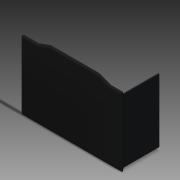
# Autodesk Inventor part: Simple3DPrintBackplate01
Saved by Autodesk Inventor 2015 (Build 190159000, 159)
## iProperties
Created: 2015-09-24
Part Number: Simple3DPrintBackplate01
Material: Aluminum 6061 Black Anodized
Document SubType Name: Modeling
Designer: -
Density: 2.71 g/cm^3
Appearance: Aluminum - Flat - Version 1.1
Author: -
Autodesk Inventor part; units mm, degrees
ref_plane "YZ Plane" through (0, 0, 0) normal (1, 0, 0) x (0, 1, 0)
ref_plane "XZ Plane" through (0, 0, 0) normal (0, 1, 0) x (-1, 0, 0)
ref_plane "XY Plane" through (0, 0, 0) normal (0, 0, 1) x (1, 0, 0)
sketch "Sketch1" plane through (0, 0, 0) normal (0, 0, 1) x (1, 0, 0)
  line L0 (25.1473, 47.4388) -> (-25.1473, 47.4388)
  line L1 (-25.8314, 47.3182) -> (-38.1686, 42.8278)
  line L2 (-38.8527, 42.7072) -> (-53.924, 42.7072)
  line L3 (-55.924, 40.7072) -> (-55.924, -28.8108)
  line L4 (-53.924, -30.8108) -> (62.994, -30.8108)
  line L5 (64.994, -28.8108) -> (64.994, 40.7072)
  line L6 (62.994, 42.7072) -> (38.8527, 42.7072)
  line L7 (38.1686, 42.8278) -> (25.8314, 47.3182)
  line L8 (0, 0) -> (0, 61.2972) construction
  arc A0 (64.994, 40.7072) -> (62.994, 42.7072) centre (62.994, 40.7072) ccw
  arc A1 (62.994, -30.8108) -> (64.994, -28.8108) centre (62.994, -28.8108) ccw
  arc A2 (-55.924, -28.8108) -> (-53.924, -30.8108) centre (-53.924, -28.8108) ccw
  arc A3 (-53.924, 42.7072) -> (-55.924, 40.7072) centre (-53.924, 40.7072) ccw
  arc A4 (-38.8527, 42.7072) -> (-38.1686, 42.8278) centre (-38.8527, 44.7072) ccw
  arc A5 (-25.1473, 47.4388) -> (-25.8314, 47.3182) centre (-25.1473, 45.4388) ccw
  arc A6 (25.8314, 47.3182) -> (25.1473, 47.4388) centre (25.1473, 45.4388) ccw
  arc A7 (38.1686, 42.8278) -> (38.8527, 42.7072) centre (38.8527, 44.7072) ccw
  point P0 (25.5, 47.4388)
  point P1 (-25.5, 47.4388)
  point P2 (-38.5, 42.7072)
  point P3 (-55.924, 42.7072)
  point P4 (-55.924, -30.8108)
  point P5 (64.994, 42.7072)
  point P6 (38.5, 42.7072)
  point P7 (0, 47.4388)
  dimension "d48" = 51
  dimension "d50" = 160
  dimension "d51" = 160
  dimension "d52" = 13
  dimension "d53" = 17.424
  dimension "d54" = 26.494
  dimension "d55" = 73.518
  dimension "d56" = 13
  dimension "d57" = 2
  constraints: 18 end point, 16 point on circle, 16 point on line, 16 tangent, 8 centre point, 7 equal radius, 4 perpendicular, 2 horizontal, 1 midpoint, 1 parallel, 1 vertical, 1 other
  measures "d48" distance of point (25.5, 47.439) point (-25.5, 47.439)
  measures "d50" angle of L0 L7
  measures "d51" angle of L0 L1
  measures "d52" horizontal distance of point (-38.5, 42.707) point (-25.5, 47.439)
  measures "d53" distance of point (-38.5, 42.707) point (-55.924, 42.707)
  measures "d54" distance of point (64.994, 42.707) point (38.5, 42.707)
  measures "d55" distance of point (-55.924, 42.707) point (-55.924, -30.811)
  measures "d56" horizontal distance of point (25.5, 47.439) point (38.5, 42.707)
  measures "d57" radius of A0
extrude "Extrusion1" add sketch "Sketch1" along normal blind 2
chamfer "Chamfer1" distance 1.5 distance2 1 16 edges at (50.9233, 42.7072, 2) (38.5054, 42.7376, 2) (32, 45.073, 2) (25.4946, 47.4084, 2) (0, 47.4388, 2) (-25.4946, 47.4084, 2) (-32, 45.073, 2) (-38.5054, 42.7376, 2) (-46.3883, 42.7072, 2) (-55.3382, 42.1214, 2) (-55.924, 5.9482, 2) (-55.3382, -30.225, 2) (4.535, -30.8108, 2) (64.4082, -30.225, 2) (64.994, 5.9482, 2) (64.4082, 42.1214, 2) measured on face at (64.0547, -29.8715, 2) measured on face at (64.0547, 41.7679, 2) measured on face at (-25.4078, 46.916, 2) measured on face at (31.829, 44.6032, 2) measured on face at (50.9233, 42.2072, 2) measured on face at (-38.4185, 42.2452, 2) measured on face at (-46.3883, 42.2072, 2) measured on face at (-55.424, 5.9482, 2) measured on face at (-31.829, 44.6032, 2) measured on face at (25.4078, 46.916, 2) measured on face at (4.535, -30.3108, 2) measured on face at (38.4185, 42.2452, 2) measured on face at (0, 46.9388, 2) measured on face at (64.494, 5.9482, 2) measured on face at (-54.9847, 41.7679, 2) measured on face at (-54.9847, -29.8715, 2)
fillet "Fillet1" radius 2 16 edges at (-54.2776, 41.0608, 2) (-46.3883, 41.2072, 2) (-38.2449, 41.2604, 2) (-31.487, 43.6635, 2) (-25.2342, 45.9312, 2) (0, 45.9388, 2) (25.2342, 45.9312, 2) (31.487, 43.6635, 2) (38.2449, 41.2604, 2) (50.9233, 41.2072, 2) (63.3476, 41.0608, 2) (63.494, 5.9482, 2) (63.3476, -29.1643, 2) (4.535, -29.3108, 2) (-54.2776, -29.1643, 2) (-54.424, 5.9482, 2)
fillet "Fillet2" radius 1 16 edges at (-55.3382, -30.225, 1) (4.535, -30.8108, 1) (64.4082, -30.225, 1) (64.994, 5.9482, 1) (64.4082, 42.1214, 1) (50.9233, 42.7072, 1) (38.5054, 42.7376, 1) (32, 45.073, 1) (25.4946, 47.4084, 1) (0, 47.4388, 1) (-25.4946, 47.4084, 1) (-32, 45.073, 1) (-38.5054, 42.7376, 1) (-46.3883, 42.7072, 1) (-55.3382, 42.1214, 1) (-55.924, 5.9482, 1)
feature "Lip1" [suppressed]
sketch "Sketch8" plane through (0, 0, 0) normal (0, 0, -1) x (-1, 0, 0)
  line L0 (-64.994, 40.7072) -> (-64.994, -28.8108) projected
  arc A0 (-64.994, -28.8108) -> (-62.994, -30.8108) centre (-62.994, -28.8108) ccw projected
  line L1 (-62.994, -30.8108) -> (53.924, -30.8108) projected
  arc A1 (53.924, -30.8108) -> (55.924, -28.8108) centre (53.924, -28.8108) ccw projected
  line L2 (55.924, -28.8108) -> (55.924, 40.7072) projected
  arc A2 (55.924, 40.7072) -> (53.924, 42.7072) centre (53.924, 40.7072) ccw projected
  line L3 (53.924, 42.7072) -> (38.8527, 42.7072) projected
  arc A3 (38.1686, 42.8278) -> (38.8527, 42.7072) centre (38.8527, 44.7072) ccw projected
  line L4 (38.1686, 42.8278) -> (25.8314, 47.3182) projected
  arc A4 (25.8314, 47.3182) -> (25.1473, 47.4388) centre (25.1473, 45.4388) ccw projected
  line L5 (25.1473, 47.4388) -> (-25.1473, 47.4388) projected
  arc A5 (-25.1473, 47.4388) -> (-25.8314, 47.3182) centre (-25.1473, 45.4388) ccw projected
  line L6 (-25.8314, 47.3182) -> (-38.1686, 42.8278) projected
  arc A6 (-38.8527, 42.7072) -> (-38.1686, 42.8278) centre (-38.8527, 44.7072) ccw projected
  line L7 (-38.8527, 42.7072) -> (-62.994, 42.7072) projected
  arc A7 (-62.994, 42.7072) -> (-64.994, 40.7072) centre (-62.994, 40.7072) ccw projected
  line L8 (-60.894, 40.6072) -> (-38.8527, 40.6072)
  arc A8 (-38.8527, 40.6072) -> (-37.4504, 40.8545) centre (-38.8527, 44.7072) ccw
  line L9 (-37.4504, 40.8545) -> (-25.7925, 45.0976)
  line L10 (-24.4244, 45.3388) -> (24.4244, 45.3388)
  line L11 (25.7925, 45.0976) -> (37.4504, 40.8545)
  arc A9 (37.4504, 40.8545) -> (38.8527, 40.6072) centre (38.8527, 44.7072) ccw
  line L12 (38.8527, 40.6072) -> (51.824, 40.6072)
  line L13 (53.824, 38.6072) -> (53.824, -26.7108)
  line L14 (51.824, -28.7108) -> (-60.894, -28.7108)
  line L15 (-62.894, -26.7108) -> (-62.894, 38.6072)
  arc A10 (-60.894, 40.6072) -> (-62.894, 38.6072) centre (-60.894, 38.6072) ccw
  arc A11 (-62.894, -26.7108) -> (-60.894, -28.7108) centre (-60.894, -26.7108) ccw
  arc A12 (51.824, -28.7108) -> (53.824, -26.7108) centre (51.824, -26.7108) ccw
  arc A13 (53.824, 38.6072) -> (51.824, 40.6072) centre (51.824, 38.6072) ccw
  arc A14 (-24.4244, 45.3388) -> (-25.7925, 45.0976) centre (-24.4244, 41.3388) ccw
  arc A15 (25.7925, 45.0976) -> (24.4244, 45.3388) centre (24.4244, 41.3388) ccw
  point P0 (0, 0)
  dimension "d62" = 2.1
  dimension "d63" = 2
  dimension "d64" = 4
  constraints: 16 end point, 16 point on circle, 12 tangent, 8 centre point, 4 equal radius, 9 other
  measures "d62" distance between parallel lines of L7 L8
  measures "d63" radius of A10
  measures "d64" radius of A14
extrude "Extrusion7" add sketch "Sketch8" along normal blind 1 contours L8 A8 L9 A14 L10 A15 L11 A9 L12 A13 L13 A12 L14 A11 L15 A10
sketch "Sketch4" plane through (0, 0, 2) normal (0, 0, 1) x (1, 0, 0)
  line L0 (92.6097, 61.0907) -> (51.0597, 61.0907)
  line L1 (51.0597, 61.0907) -> (51.0597, -62.6292)
  line L2 (51.0597, -62.6292) -> (92.6097, -62.6292)
  line L3 (92.6097, -62.6292) -> (92.6097, 61.0907)
  line L4 (64.5487, 40.7072) -> (64.5487, -28.8108) projected
  point P0 (0, 0)
  dimension "d21" = 123.7199
  dimension "d22" = 41.55
  dimension "d58" = 13.489
  constraints: 8 end point, 2 parallel, 1 horizontal, 1 perpendicular
  measures "d21" distance between parallel lines of L2 L0
  measures "d22" distance between parallel lines of L3 L1
  measures "d58" distance between parallel lines of L1 L4
extrude "Extrusion3" cut sketch "Sketch4" against normal blind 10
sketch "Sketch7" plane through (0, 0, 0) normal (0, 0, -1) x (-1, 0, 0)
  line L0 (-51.0597, 39.6572) -> (-49.7257, 39.6572)
  line L1 (-49.7257, 39.6572) -> (-49.7257, -27.7608)
  line L2 (-49.7257, -27.7608) -> (-51.0597, -27.7608)
  line L3 (-51.0597, -27.7608) -> (-51.0597, 39.6572)
  line L4 (-51.0597, -28.7108) -> (-51.0597, -30.8108) projected
  line L5 (53.924, -30.8108) -> (-51.0597, -30.8108) projected
  line L6 (-51.0597, 42.7072) -> (-38.8527, 42.7072) projected
  point P0 (0, 0)
  point P1 (-51.0597, -28.8108)
  point P2 (-51.0597, 40.7072)
  point P3 (-32.4217, 42.6092)
  dimension "d35" = 1.334
  dimension "d59" = 3.05
  dimension "d60" = 3.05
  dimension "d61" = 67.418
  constraints: 8 end point, 2 parallel, 1 horizontal, 1 perpendicular, 1 vertical, 1 other
  measures "d35" distance between parallel lines of L3 L1
  measures "d59" distance between parallel lines of L5 L2
  measures "d60" distance between parallel lines of L0 L6
  measures "d61" distance between parallel lines of L2 L0
extrude "Extrusion6" add sketch "Sketch7" along normal blind 39
body "Solid1"
